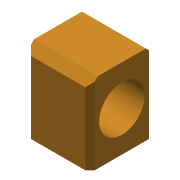
# Autodesk Inventor part: 3136 1094 56
Saved by Autodesk Inventor 2022 Beta2 (Build 260130000, 130) ContinuousBuild 0
## iProperties
Shininess: 64.0
Length Units: 11269
Angle Units: 11279
Time Units: 11290
Mass Units: 11283
Length Display Precision: 3
Angle Display Precision: 2
Compacted: True
Part Number: 3136 1094 56
Document SubType Name: Modeling
Created: 2003-04-13
Designer: Uffe Bak
Material: Steel, Mild
Density: 7.86 g/cm^3
Appearance: Brokk-Gul
Density: 0.0
Volumn: 0.0
Area: 0.0
PropertySet Name: Model Information
Control State: 0
Master: False
Checked Out: False
Author: Uffe Bak
Autodesk Inventor part; units mm, degrees
ref_plane "YZ Plane" through (0, 0, 0) normal (1, 0, 0) x (0, 1, 0)
ref_plane "XZ Plane" through (0, 0, 0) normal (0, 1, 0) x (-1, 0, 0)
ref_plane "XY Plane" through (0, 0, 0) normal (0, 0, 1) x (1, 0, 0)
sketch "Sketch1" plane through (0, 0, 0) normal (0, 0, 1) x (1, 0, 0)
  line L0 (40, 40) -> (40, -40)
  line L1 (40, -40) -> (-40, -40)
  line L2 (-40, -40) -> (-40, 40)
  line L3 (-40, 40) -> (40, 40)
  point P0 (0, 0)
  point P1 (0, 0)
  dimension "d0" = 80
  constraints: 8 end point, 1 coincident, 7 other
  measures "d0" distance of L2.end L0.start
extrude "Extrusion1" add sketch "Sketch1" along normal blind 100
sketch "Sketch2" plane through (-40, -40, 0) normal (-1, 0, 0) x (0, 0, 1)
  line L0 (100, 0) -> (100, 80) projected
  line L1 (0, 80) -> (100, 80) projected
  point P0 (50, 40)
  dimension "d3" = 50
  dimension "d4" = 40
  measures "d3" distance from line of L0 point (50, 40)
  measures "d4" distance from line of L1 point (50, 40)
hole "Hole1" at (-40, 0, 50) direction (1, 0, 0) diameter 57 end through all
chamfer "Chamfer2" distance 10 angle 45 2 edges at (0, -40, 100) (0, 40, 100)
chamfer "Chamfer1" distance 6 angle 45 4 edges at (-40, 40, 45) (40, 40, 45) (-40, -40, 45) (40, -40, 45)
body "Solid1"
